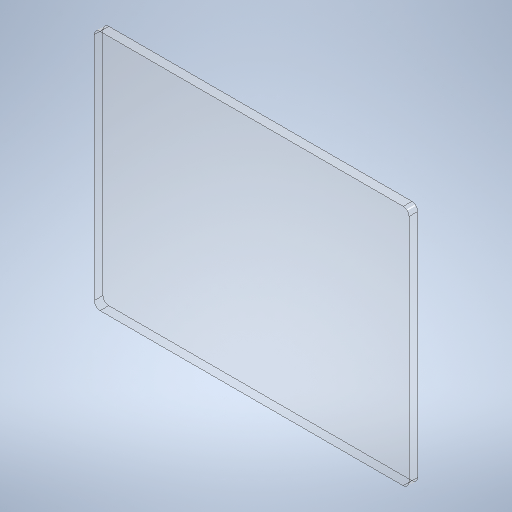
# Autodesk Inventor part: Tampa
Saved by Autodesk Inventor 2025 (Build 290162000, 162)
## iProperties
Created: 2024-10-12
Part Number: Tampa
Material: PMMA plástico
Document SubType Name: Modeling
Designer: Andre
Density: 1.188 g/cm^3
Appearance: Policarbonato - Transparente
Author: Andre
Autodesk Inventor part; units mm, degrees
ref_plane "YZ Plane" through (0, 0, 0) normal (1, 0, 0) x (0, 1, 0)
ref_plane "XZ Plane" through (0, 0, 0) normal (0, 1, 0) x (-1, 0, 0)
ref_plane "XY Plane" through (0, 0, 0) normal (0, 0, 1) x (1, 0, 0)
sketch "Esboço1" plane through (0, 0, 0) normal (0, 0, 1) x (1, 0, 0)
  line L0 (-54, -41.5) -> (54, -41.5)
  line L1 (54, -41.5) -> (54, 41.5)
  line L2 (54, 41.5) -> (-54, 41.5)
  line L3 (-54, 41.5) -> (-54, -41.5)
  line L4 (-54, -41.5) -> (54, 41.5) construction
  line L5 (54, -41.5) -> (-54, 41.5) construction
  point P0 (0, 0)
  dimension "d0" = 108
  dimension "d1" = 83
  constraints: 12 end point, 2 midpoint, 2 parallel, 1 horizontal, 1 perpendicular
  measures "d0" distance of L2.end L1.end
  measures "d1" distance of L1.end L0.end
extrude "Extrusão1" add sketch "Esboço1" along normal blind 3
fillet "Arredondamento1" radius 2 4 edges at (54, 41.5, 1.5) (-54, 41.5, 1.5) (54, -41.5, 1.5) (-54, -41.5, 1.5)
